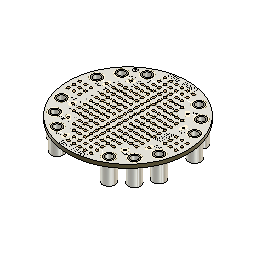
4320 PermaProto Gizmo (Autodesk Fusion 360 design; units mm, degrees)
part number: FIDUCIAL_1MM
part number: SEWTAP_SMTNUTM3
Autodesk Fusion 360 part; units mm, degrees
sketch "sketch 305" plane through (0, 0, 0) normal (0, 0, 1) x (1, 0, 0)
  circle A0 centre (0, 0) radius 26.67
extrude "Board" add sketch "sketch 305" along normal blind 1.57 makes body 1 in component "Board"
sketch "sketch 1798" plane through (0, 0, 0) normal (0, 0, 1) x (1, 0, 0)
  line L0 (-0.75, -0.75) -> (0.75, -0.75)
  line L1 (0.75, -0.75) -> (0.75, 0.75)
  line L2 (0.75, 0.75) -> (-0.75, 0.75)
  line L3 (-0.75, 0.75) -> (-0.75, -0.75)
extrude "FIDUCIAL_1MM" add sketch "sketch 1798" along normal blind 0.1 separate body makes body 2 in component "FIDUCIAL_1MM"
sketch "sketch 1933" plane through (0, 0, 0) normal (0, 0, 1) x (1, 0, 0)
  line L0 (-0.898, -0.898) -> (0.898, -0.898)
  line L1 (0.898, -0.898) -> (0.898, 0.898)
  line L2 (0.898, 0.898) -> (-0.898, 0.898)
  line L3 (-0.898, 0.898) -> (-0.898, -0.898)
extrude "PCBFEAT-REV-040" add sketch "sketch 1933" along normal blind 0.1 separate body makes body 3 in component "PCBFEAT-REV-040"
sketch "sketch 2156" plane through (0, 0, 0) normal (0, 0, 1) x (1, 0, 0)
  line L0 (-2.667, -2.667) -> (2.667, -2.667)
  line L1 (2.667, -2.667) -> (2.667, 2.667)
  line L2 (2.667, 2.667) -> (-2.667, 2.667)
  line L3 (-2.667, 2.667) -> (-2.667, -2.667)
extrude "SMT_NUT_3MM" add sketch "sketch 2156" along normal blind 0.1 separate body makes body 4 in component "SMT_NUT_3MM"
sketch "sketch 2355" plane through (0, 0, 0) normal (0, 0, 1) x (1, 0, 0)
  line L0 (-0.5, -0.5) -> (0.5, -0.5)
  line L1 (0.5, -0.5) -> (0.5, 0.5)
  line L2 (0.5, 0.5) -> (-0.5, 0.5)
  line L3 (-0.5, 0.5) -> (-0.5, -0.5)
extrude "1X01_OVAL" add sketch "sketch 2355" along normal blind 0.1 separate body makes body 5 in component "1X01_OVAL"
sketch "sketch 397" plane through (0, 0, 0) normal (0, 0, 1) x (1, 0, 0)
  circle A0 centre (1.27, 17.78) radius 0.6
  circle A1 centre (1.27, 15.24) radius 0.6
  circle A2 centre (1.27, 12.7) radius 0.6
  circle A3 centre (1.27, 10.16) radius 0.6
  circle A4 centre (1.27, 7.62) radius 0.6
  circle A5 centre (1.27, 5.08) radius 0.6
  circle A6 centre (1.27, 0) radius 0.6
  circle A7 centre (1.27, 2.54) radius 0.6
  circle A8 centre (1.27, -2.54) radius 0.6
  circle A9 centre (1.27, -5.08) radius 0.6
  circle A10 centre (1.27, -7.62) radius 0.6
  circle A11 centre (1.27, -10.16) radius 0.6
  circle A12 centre (1.27, -12.7) radius 0.6
  circle A13 centre (1.27, -15.24) radius 0.6
  circle A14 centre (1.27, -17.78) radius 0.6
  circle A15 centre (-1.27, 17.78) radius 0.6
  circle A16 centre (-1.27, 15.24) radius 0.6
  circle A17 centre (-1.27, 12.7) radius 0.6
  circle A18 centre (-1.27, 10.16) radius 0.6
  circle A19 centre (-1.27, 7.62) radius 0.6
  circle A20 centre (-1.27, 5.08) radius 0.6
  circle A21 centre (-1.27, 0) radius 0.6
  circle A22 centre (-1.27, 2.54) radius 0.6
  circle A23 centre (-1.27, -2.54) radius 0.6
  circle A24 centre (-1.27, -5.08) radius 0.6
  circle A25 centre (-1.27, -7.62) radius 0.6
  circle A26 centre (-1.27, -10.16) radius 0.6
  circle A27 centre (-1.27, -12.7) radius 0.6
  circle A28 centre (-1.27, -15.24) radius 0.6
  circle A29 centre (-1.27, -17.78) radius 0.6
  circle A30 centre (3.81, -17.78) radius 0.6
  circle A31 centre (6.35, -17.78) radius 0.6
  circle A32 centre (8.89, -15.24) radius 0.6
  circle A33 centre (6.35, -15.24) radius 0.6
  circle A34 centre (3.81, -15.24) radius 0.6
  circle A35 centre (8.89, -12.7) radius 0.6
  circle A36 centre (6.35, -12.7) radius 0.6
  circle A37 centre (3.81, -12.7) radius 0.6
  circle A38 centre (13.97, -10.16) radius 0.6
  circle A39 centre (11.43, -10.16) radius 0.6
  circle A40 centre (8.89, -10.16) radius 0.6
  circle A41 centre (6.35, -10.16) radius 0.6
  circle A42 centre (3.81, -10.16) radius 0.6
  circle A43 centre (13.97, -7.62) radius 0.6
  circle A44 centre (11.43, -7.62) radius 0.6
  circle A45 centre (8.89, -7.62) radius 0.6
  circle A46 centre (6.35, -7.62) radius 0.6
  circle A47 centre (3.81, -7.62) radius 0.6
  circle A48 centre (13.97, -5.08) radius 0.6
  circle A49 centre (11.43, -5.08) radius 0.6
  circle A50 centre (8.89, -5.08) radius 0.6
  circle A51 centre (6.35, -5.08) radius 0.6
  circle A52 centre (3.81, -5.08) radius 0.6
  circle A53 centre (13.97, 0) radius 0.6
  circle A54 centre (11.43, 0) radius 0.6
  circle A55 centre (8.89, 0) radius 0.6
  circle A56 centre (6.35, 0) radius 0.6
  circle A57 centre (3.81, 0) radius 0.6
  circle A58 centre (13.97, -2.54) radius 0.6
  circle A59 centre (11.43, -2.54) radius 0.6
  circle A60 centre (8.89, -2.54) radius 0.6
  circle A61 centre (6.35, -2.54) radius 0.6
  circle A62 centre (3.81, -2.54) radius 0.6
  circle A63 centre (13.97, 2.54) radius 0.6
  circle A64 centre (11.43, 2.54) radius 0.6
  circle A65 centre (8.89, 2.54) radius 0.6
  circle A66 centre (6.35, 2.54) radius 0.6
  circle A67 centre (3.81, 2.54) radius 0.6
  circle A68 centre (13.97, 5.08) radius 0.6
  circle A69 centre (11.43, 5.08) radius 0.6
  circle A70 centre (8.89, 5.08) radius 0.6
  circle A71 centre (6.35, 5.08) radius 0.6
  circle A72 centre (3.81, 5.08) radius 0.6
  circle A73 centre (13.97, 7.62) radius 0.6
  circle A74 centre (11.43, 7.62) radius 0.6
  circle A75 centre (8.89, 7.62) radius 0.6
  circle A76 centre (6.35, 7.62) radius 0.6
  circle A77 centre (3.81, 7.62) radius 0.6
  circle A78 centre (13.97, 10.16) radius 0.6
  circle A79 centre (11.43, 10.16) radius 0.6
  circle A80 centre (8.89, 10.16) radius 0.6
  circle A81 centre (6.35, 10.16) radius 0.6
  circle A82 centre (3.81, 10.16) radius 0.6
  circle A83 centre (8.89, 12.7) radius 0.6
  circle A84 centre (6.35, 12.7) radius 0.6
  circle A85 centre (3.81, 12.7) radius 0.6
  circle A86 centre (8.89, 15.24) radius 0.6
  circle A87 centre (6.35, 15.24) radius 0.6
  circle A88 centre (3.81, 15.24) radius 0.6
  circle A89 centre (6.35, 17.78) radius 0.6
  circle A90 centre (3.81, 17.78) radius 0.6
  circle A91 centre (-6.35, 17.78) radius 0.6
  circle A92 centre (-3.81, 17.78) radius 0.6
  circle A93 centre (-8.89, 12.7) radius 0.6
  circle A94 centre (-6.35, 12.7) radius 0.6
  circle A95 centre (-3.81, 12.7) radius 0.6
  circle A96 centre (-8.89, 15.24) radius 0.6
  circle A97 centre (-6.35, 15.24) radius 0.6
  circle A98 centre (-3.81, 15.24) radius 0.6
  circle A99 centre (-13.97, 10.16) radius 0.6
  circle A100 centre (-11.43, 10.16) radius 0.6
  circle A101 centre (-8.89, 10.16) radius 0.6
  circle A102 centre (-6.35, 10.16) radius 0.6
  circle A103 centre (-3.81, 10.16) radius 0.6
  circle A104 centre (-13.97, 7.62) radius 0.6
  circle A105 centre (-11.43, 7.62) radius 0.6
  circle A106 centre (-8.89, 7.62) radius 0.6
  circle A107 centre (-6.35, 7.62) radius 0.6
  circle A108 centre (-3.81, 7.62) radius 0.6
  circle A109 centre (-13.97, 2.54) radius 0.6
  circle A110 centre (-11.43, 2.54) radius 0.6
  circle A111 centre (-8.89, 2.54) radius 0.6
  circle A112 centre (-6.35, 2.54) radius 0.6
  circle A113 centre (-3.81, 2.54) radius 0.6
  circle A114 centre (-13.97, 5.08) radius 0.6
  circle A115 centre (-11.43, 5.08) radius 0.6
  circle A116 centre (-8.89, 5.08) radius 0.6
  circle A117 centre (-6.35, 5.08) radius 0.6
  circle A118 centre (-3.81, 5.08) radius 0.6
  circle A119 centre (-13.97, 0) radius 0.6
  circle A120 centre (-11.43, 0) radius 0.6
  circle A121 centre (-8.89, 0) radius 0.6
  circle A122 centre (-3.81, 0) radius 0.6
  circle A123 centre (-6.35, 0) radius 0.6
  circle A124 centre (-13.97, -2.54) radius 0.6
  circle A125 centre (-11.43, -2.54) radius 0.6
  circle A126 centre (-8.89, -2.54) radius 0.6
  circle A127 centre (-6.35, -2.54) radius 0.6
  circle A128 centre (-3.81, -2.54) radius 0.6
  circle A129 centre (-13.97, -5.08) radius 0.6
  circle A130 centre (-11.43, -5.08) radius 0.6
  circle A131 centre (-8.89, -5.08) radius 0.6
  circle A132 centre (-6.35, -5.08) radius 0.6
  circle A133 centre (-3.81, -5.08) radius 0.6
  circle A134 centre (-13.97, -7.62) radius 0.6
  circle A135 centre (-11.43, -7.62) radius 0.6
  circle A136 centre (-8.89, -7.62) radius 0.6
  circle A137 centre (-6.35, -7.62) radius 0.6
  circle A138 centre (-3.81, -7.62) radius 0.6
  circle A139 centre (-8.89, -12.7) radius 0.6
  circle A140 centre (-6.35, -12.7) radius 0.6
  circle A141 centre (-3.81, -12.7) radius 0.6
  circle A142 centre (-13.97, -10.16) radius 0.6
  circle A143 centre (-11.43, -10.16) radius 0.6
  circle A144 centre (-8.89, -10.16) radius 0.6
  circle A145 centre (-6.35, -10.16) radius 0.6
  circle A146 centre (-3.81, -10.16) radius 0.6
  circle A147 centre (-8.89, -15.24) radius 0.6
  circle A148 centre (-6.35, -15.24) radius 0.6
  circle A149 centre (-3.81, -15.24) radius 0.6
  circle A150 centre (-6.35, -17.78) radius 0.6
  circle A151 centre (-3.81, -17.78) radius 0.6
  circle A152 centre (-3.81, -20.32) radius 0.6
  circle A153 centre (-3.81, -22.86) radius 0.6
  circle A154 centre (-1.27, -22.86) radius 0.6
  circle A155 centre (-1.27, -20.32) radius 0.6
  circle A156 centre (1.27, -20.32) radius 0.6
  circle A157 centre (1.27, -22.86) radius 0.6
  circle A158 centre (3.81, -22.86) radius 0.6
  circle A159 centre (3.81, -20.32) radius 0.6
  circle A160 centre (6.35, -20.32) radius 0.6
  circle A161 centre (6.35, -22.86) radius 0.6
  circle A162 centre (-6.35, 20.32) radius 0.6
  circle A163 centre (-3.81, 20.32) radius 0.6
  circle A164 centre (-3.81, 22.86) radius 0.6
  circle A165 centre (-6.35, 22.86) radius 0.6
  circle A166 centre (6.35, 20.32) radius 0.6
  circle A167 centre (3.81, 20.32) radius 0.6
  circle A168 centre (3.81, 22.86) radius 0.6
  circle A169 centre (1.27, 22.86) radius 0.6
  circle A170 centre (1.27, 20.32) radius 0.6
  circle A171 centre (-1.27, 20.32) radius 0.6
  circle A172 centre (-1.27, 22.86) radius 0.6
  circle A173 centre (6.35, 22.86) radius 0.6
  circle A174 centre (19.05, -2.54) radius 0.6
  circle A175 centre (19.05, 2.54) radius 0.6
  circle A176 centre (19.05, 0) radius 0.6
  circle A177 centre (21.59, 2.54) radius 0.6
  circle A178 centre (21.59, 0) radius 0.6
  circle A179 centre (21.59, -2.54) radius 0.6
  circle A180 centre (24.13, -2.54) radius 0.6
  circle A181 centre (24.13, 0) radius 0.6
  circle A182 centre (24.13, 2.54) radius 0.6
  circle A183 centre (-19.05, -2.54) radius 0.6
  circle A184 centre (-19.05, 0) radius 0.6
  circle A185 centre (-19.05, 2.54) radius 0.6
  circle A186 centre (-21.59, 2.54) radius 0.6
  circle A187 centre (-24.13, 2.54) radius 0.6
  circle A188 centre (-24.13, 0) radius 0.6
  circle A189 centre (-21.59, 0) radius 0.6
  circle A190 centre (-21.59, -2.54) radius 0.6
  circle A191 centre (-24.13, -2.54) radius 0.6
  circle A192 centre (-11.557, 20.117) radius 2.125
  circle A193 centre (-11.557, -20.117) radius 2.125
  circle A194 centre (11.557, 20.117) radius 2.125
  circle A195 centre (11.557, -20.117) radius 2.125
  circle A196 centre (-17.78, 14.935) radius 2.125
  circle A197 centre (-21.819, 7.925) radius 2.125
  circle A198 centre (-21.819, -7.925) radius 2.125
  circle A199 centre (-17.78, -14.935) radius 2.125
  circle A200 centre (17.78, 14.935) radius 2.125
  circle A201 centre (21.819, 7.925) radius 2.125
  circle A202 centre (21.819, -7.925) radius 2.125
  circle A203 centre (17.78, -14.935) radius 2.125
  circle A204 centre (12.7, -13.97) radius 0.5
  circle A205 centre (17.145, -7.62) radius 0.5
  circle A206 centre (17.145, 7.62) radius 0.5
  circle A207 centre (12.7, 13.97) radius 0.5
  circle A208 centre (-12.7, -13.97) radius 0.5
  circle A209 centre (-17.145, -7.62) radius 0.5
  circle A210 centre (-17.145, 7.62) radius 0.5
  circle A211 centre (-12.7, 13.97) radius 0.5
  circle A212 centre (-6.35, -21.59) radius 0.5
extrude "Extrude2" cut sketch "sketch 397" along normal blind 1.57 bodies 1 in component "Board"
sketch "Sketch1" plane through (0, 0, 1.57) normal (0, 0, 1) x (-1, 0, 0) in component "Component"
  circle A0 centre (11.557, -20.117) radius 2.125
  circle A1 centre (17.78, -14.935) radius 2.125
  circle A2 centre (21.819, -7.925) radius 2.125
  circle A3 centre (21.819, 7.925) radius 2.125
  circle A4 centre (17.78, 14.935) radius 2.125
  circle A5 centre (11.557, 20.117) radius 2.125
  circle A6 centre (-11.557, 20.117) radius 2.125
  circle A7 centre (-17.78, 14.935) radius 2.125
  circle A8 centre (-21.819, 7.925) radius 2.125
  circle A9 centre (-21.819, -7.925) radius 2.125
  circle A10 centre (-17.78, -14.935) radius 2.125
  circle A11 centre (-11.557, -20.117) radius 2.125
  circle A12 centre (11.557, -20.117) radius 2.75
  circle A13 centre (11.557, -20.117) radius 1.5
  circle A14 centre (17.78, -14.935) radius 1.5
  circle A15 centre (17.78, -14.935) radius 2.75
  circle A16 centre (21.819, -7.925) radius 2.75
  circle A17 centre (21.819, -7.925) radius 1.5
  circle A18 centre (21.819, 7.925) radius 1.5
  circle A19 centre (21.819, 7.925) radius 2.75
  circle A20 centre (17.78, 14.935) radius 1.5
  circle A21 centre (17.78, 14.935) radius 2.75
  circle A22 centre (11.557, 20.117) radius 1.5
  circle A23 centre (11.557, 20.117) radius 2.75
  circle A24 centre (-11.557, 20.117) radius 1.5
  circle A25 centre (-11.557, 20.117) radius 2.75
  circle A26 centre (-17.78, 14.935) radius 1.5
  circle A27 centre (-17.78, 14.935) radius 2.75
  circle A28 centre (-21.819, 7.925) radius 1.5
  circle A29 centre (-21.819, 7.925) radius 2.75
  circle A30 centre (-21.819, -7.925) radius 2.75
  circle A31 centre (-21.819, -7.925) radius 1.5
  circle A32 centre (-11.557, -20.117) radius 1.5
  circle A33 centre (-11.557, -20.117) radius 2.75
  circle A34 centre (-17.78, -14.935) radius 1.5
  circle A35 centre (-17.78, -14.935) radius 2.75
  dimension "d14" = 5.5
  dimension "d15" = 3
  dimension "d17" = 3
  dimension "d18" = 5.5
  dimension "d19" = 5.5
  dimension "d20" = 3
  dimension "d25" = 3
  dimension "d26" = 5.5
  dimension "d27" = 3
  dimension "d28" = 5.5
  dimension "d29" = 3
  dimension "d30" = 5.5
  dimension "d31" = 3
  dimension "d32" = 5.5
  dimension "d33" = 3
  dimension "d34" = 5.5
  dimension "d35" = 3
  dimension "d36" = 5.5
  dimension "d37" = 5.5
  dimension "d38" = 3
  dimension "d39" = 3
  dimension "d40" = 5.5
  dimension "d41" = 3
  dimension "d42" = 5.5
  constraint concentric A0 A12
  constraint concentric A12 A13
  constraint concentric A1 A14
  constraint concentric A14 A15
  constraint concentric A2 A16
  constraint concentric A2 A17
  constraint concentric A3 A18
  constraint concentric A3 A19
  constraint concentric A4 A20
  constraint concentric A20 A21
  constraint concentric A5 A22
  constraint concentric A5 A23
  constraint concentric A6 A24
  constraint concentric A24 A25
  constraint concentric A7 A26
  constraint concentric A7 A27
  constraint concentric A8 A28
  constraint concentric A28 A29
  constraint concentric A9 A30
  constraint concentric A9 A31
  constraint concentric A11 A32
  constraint concentric A11 A33
  constraint concentric A10 A34
  constraint concentric A10 A35
  measures "d14" diameter of A12
  measures "d15" diameter of A13
  measures "d17" diameter of A14
  measures "d18" diameter of A15
  measures "d19" diameter of A16
  measures "d20" diameter of A17
  measures "d25" diameter of A18
  measures "d26" diameter of A19
  measures "d27" diameter of A20
  measures "d28" diameter of A21
  measures "d29" diameter of A22
  measures "d30" diameter of A23
  measures "d31" diameter of A24
  measures "d32" diameter of A25
  measures "d33" diameter of A26
  measures "d34" diameter of A27
  measures "d35" diameter of A28
  measures "d36" diameter of A29
  measures "d37" diameter of A30
  measures "d38" diameter of A31
  measures "d39" diameter of A32
  measures "d40" diameter of A33
  measures "d41" diameter of A34
  measures "d42" diameter of A35
extrude "Extrude1" add sketch "Sketch1" against normal blind 1.6 separate body contours A0 | A1 | A2 | A3 | A4 | A5 | A6 | A7 | A8 | A9 | A10 | A11 makes body 6 at (-13.6794, 20.2229, 0.5033) makes body 7 at (-19.9024, 15.0409, 0.5033) makes body 8 at (-23.9414, 8.0309, 0.5033) makes body 9 at (-23.9414, -7.8191, 0.5033) makes body 10 at (19.6966, 8.0309, 0.5033) makes body 11 at (19.6966, -7.8191, 0.5033) makes body 12 at (-19.9024, -14.8291, 0.5033) makes body 13 at (9.4346, -20.0111, 0.5033) makes body 14 at (15.6576, 15.0409, 0.5033) makes body 15 at (9.4346, 20.2229, 0.5033) makes body 16 at (15.6576, -14.8291, 0.5033) makes body 17 at (-13.6794, -20.0111, 0.5033) in component "Component"
extrude "Extrude2'" add sketch "Sketch1" against normal blind 8 from surface at -1.6 contours A0 | A1 | A2 | A3 | A4 | A5 | A6 | A7 | A8 | A9 | A10 | A11 | A12 | A15 | A16 | A19 | A21 | A23 | A25 | A27 | A29 | A30 | A33 | A35 bodies 9 10 7 8 11 12 13 14 6 15 16 17 in component "Component"
component "PCB Component" placed x (1, 0, 0) y (0, 1, 0) z (0, 0, 1) at (0, 0, 0)
component "Board" placed x (1, 0, 0) y (0, 1, 0) z (0, 0, 1) at (0, 0, 0) in component "PCB Component"
component "FIDUCIAL_1MM" placed x (-1, 0, 0) y (0, 1, 0) z (0, 0, -1) at (16.129, 19.177, 0) in component "PCB Component"
component "FIDUCIAL_1MM" placed x (-1, 0, 0) y (0, 1, 0) z (0, 0, -1) at (-16.002, -19.177, 0) in component "PCB Component"
component "PCBFEAT-REV-040" placed x (1, 0, 0) y (0, 1, 0) z (0, 0, 1) at (-16.002, 19.304, 1.57) in component "PCB Component"
component "SMT_NUT_3MM" placed x (0, 1, 0) y (1, 0, 0) z (0, 0, -1) at (-11.557, 20.117, 0) in component "PCB Component"
component "SMT_NUT_3MM" placed x (0, 1, 0) y (1, 0, 0) z (0, 0, -1) at (-11.557, -20.117, 0) in component "PCB Component"
component "SMT_NUT_3MM" placed x (0, 1, 0) y (1, 0, 0) z (0, 0, -1) at (11.557, 20.117, 0) in component "PCB Component"
component "SMT_NUT_3MM" placed x (0, 1, 0) y (1, 0, 0) z (0, 0, -1) at (11.557, -20.117, 0) in component "PCB Component"
component "SMT_NUT_3MM" placed x (0, 1, 0) y (1, 0, 0) z (0, 0, -1) at (-17.78, 14.935, 0) in component "PCB Component"
component "SMT_NUT_3MM" placed x (0, 1, 0) y (1, 0, 0) z (0, 0, -1) at (-21.819, 7.925, 0) in component "PCB Component"
component "SMT_NUT_3MM" placed x (0, 1, 0) y (1, 0, 0) z (0, 0, -1) at (-21.819, -7.925, 0) in component "PCB Component"
component "SMT_NUT_3MM" placed x (0, 1, 0) y (1, 0, 0) z (0, 0, -1) at (-17.78, -14.935, 0) in component "PCB Component"
component "SMT_NUT_3MM" placed x (0, 1, 0) y (1, 0, 0) z (0, 0, -1) at (17.78, 14.935, 0) in component "PCB Component"
component "SMT_NUT_3MM" placed x (0, 1, 0) y (1, 0, 0) z (0, 0, -1) at (21.819, 7.925, 0) in component "PCB Component"
component "SMT_NUT_3MM" placed x (0, 1, 0) y (1, 0, 0) z (0, 0, -1) at (21.819, -7.925, 0) in component "PCB Component"
component "SMT_NUT_3MM" placed x (0, 1, 0) y (1, 0, 0) z (0, 0, -1) at (17.78, -14.935, 0) in component "PCB Component"
component "1X01_OVAL" placed x (-0.707107, 0.707107, 0) y (-0.707107, -0.707107, 0) z (0, 0, 1) at (12.7, -13.97, 1.57) in component "PCB Component"
component "1X01_OVAL" placed x (1, 0, 0) y (0, 1, 0) z (0, 0, 1) at (17.145, -7.62, 1.57) in component "PCB Component"
component "1X01_OVAL" placed x (1, 0, 0) y (0, 1, 0) z (0, 0, 1) at (17.145, 7.62, 1.57) in component "PCB Component"
component "1X01_OVAL" placed x (0.707107, 0.707107, 0) y (-0.707107, 0.707107, 0) z (0, 0, 1) at (12.7, 13.97, 1.57) in component "PCB Component"
component "1X01_OVAL" placed x (0.707107, 0.707107, 0) y (-0.707107, 0.707107, 0) z (0, 0, 1) at (-12.7, -13.97, 1.57) in component "PCB Component"
component "1X01_OVAL" placed x (1, 0, 0) y (0, 1, 0) z (0, 0, 1) at (-17.145, -7.62, 1.57) in component "PCB Component"
component "1X01_OVAL" placed x (1, 0, 0) y (0, 1, 0) z (0, 0, 1) at (-17.145, 7.62, 1.57) in component "PCB Component"
component "1X01_OVAL" placed x (0.707107, -0.707107, 0) y (0.707107, 0.707107, 0) z (0, 0, 1) at (-12.7, 13.97, 1.57) in component "PCB Component"
component "1X01_OVAL" placed x (1, 0, 0) y (0, 1, 0) z (0, 0, 1) at (-6.35, -21.59, 1.57) in component "PCB Component"
component "Component" placed x (1, 0, 0) y (0, 1, 0) z (0, 0, 1) at (0, 0, 0) in component "PCB Component"
named bodies: "Board", "FIDUCIAL_1MM", "PCBFEAT-REV-040", "SMT_NUT_3MM", "1X01_OVAL"
